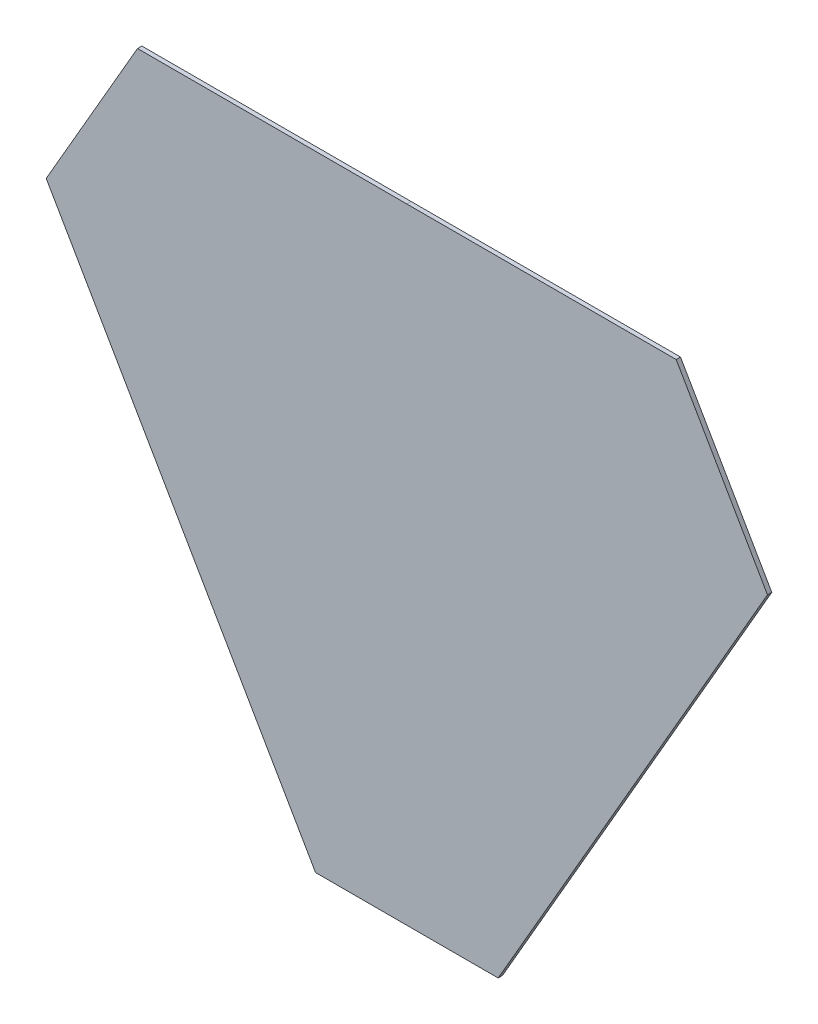
# Autodesk Inventor part: glass
Saved by Autodesk Inventor 2016 SP1 (Build 200210100, 210)
## iProperties
Created: 2016-04-18
Part Number: glass
Material: Glass
Document SubType Name: Modeling
Designer: ubik
Density: 2.18 g/cm^3
Appearance: Clear - Blue
Author: ubik
Autodesk Inventor part; units mm, degrees
ref_plane "YZ Plane" through (0, 0, 0) normal (1, 0, 0) x (0, 1, 0)
ref_plane "XZ Plane" through (0, 0, 0) normal (0, 1, 0) x (-1, 0, 0)
ref_plane "XY Plane" through (0, 0, 0) normal (0, 0, 1) x (1, 0, 0)
sketch "Sketch1" plane through (0, 0, 0) normal (0, 0, 1) x (1, 0, 0)
  line L0 (250.9966, 205.3522) -> (187.4463, 315.4245)
  line L1 (187.4463, 315.4245) -> (-0.0002, 315.4245)
  line L2 (157.2736, 43.0193) -> (250.9966, 205.3522)
  line L3 (-63.5502, -119.3142) -> (63.5503, -119.3142)
  line L4 (63.5503, -119.3142) -> (157.2736, 43.0193)
  line L5 (-157.2732, 43.0188) -> (-63.5502, -119.3142)
  line L6 (-187.4461, 315.4245) -> (-250.9964, 205.3523)
  line L7 (-250.9964, 205.3523) -> (-157.2732, 43.0188)
  line L8 (-0.0002, 315.4245) -> (-187.4461, 315.4245)
  constraints: 18 end point
extrude "Extrusion1" add sketch "Sketch1" along normal blind 3
body "Solid1"
